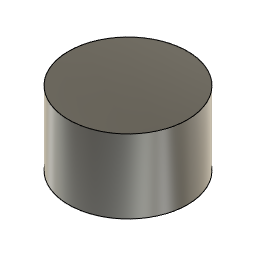
whole assembly (Autodesk Fusion 360 archive; units mm, degrees)
design "Knob"
Autodesk Fusion 360 part; units mm, degrees
(part 1 of 4)
sketch "Sketch1" plane through (0, 0, 0) normal (0, 0, 1) x (1, 0, 0)
  circle A0 centre (0, 0) radius 12.5
  circle A1 centre (0, 0) radius 3
  dimension "d1" = 25
  dimension "d2" = 6
  constraint coincident A0.centre A1.centre
  measures "d1" diameter of A0
  measures "d2" diameter of A1
extrude "Extrude1" add sketch "Sketch1" along normal blind 15.5 contours A0 | A1
extrude "Extrude2" cut sketch "Sketch1" along normal blind 11 contours A1

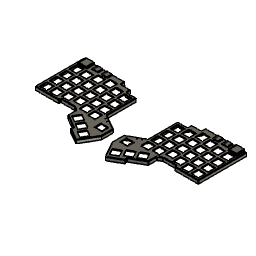
design "both_frame"
Autodesk Fusion 360 part; units mm, degrees
sketch "Sketch2" plane through (0, 0, 0) normal (0, 0, 1) x (1, 0, 0)
  line L0 (30.0248, 56.3298) -> (68.0248, 56.3298) construction
  line L1 (68.0248, 56.3298) -> (68.0248, -19.6702) construction
  line L2 (68.0248, -19.6702) -> (30.0248, -19.6702) construction
  line L3 (30.0248, -19.6702) -> (30.0248, 56.3298) construction
  line L4 (11.0248, 60.3298) -> (30.0248, 60.3298) construction
  line L5 (30.0248, 60.3298) -> (30.0248, -15.6702) construction
  line L6 (30.0248, -15.6702) -> (11.0248, -15.6702) construction
  line L7 (11.0248, -15.6702) -> (11.0248, 60.3298) construction
  line L8 (-7.9752, 64.3298) -> (11.0248, 64.3298) construction
  line L9 (11.0248, 64.3298) -> (11.0248, -11.6702) construction
  line L10 (11.0248, -11.6702) -> (-7.9752, -11.6702) construction
  line L11 (-7.9752, -11.6702) -> (-7.9752, 64.3298) construction
  line L12 (-26.9752, -18.6702) -> (-7.9752, -18.6702) construction
  line L13 (-7.9752, -18.6702) -> (-7.9752, 57.3298) construction
  line L14 (-7.9752, 57.3298) -> (-26.9752, 57.3298) construction
  line L15 (-26.9752, 57.3298) -> (-26.9752, -18.6702) construction
  line L16 (-45.9752, -21.6702) -> (-26.9752, -21.6702) construction
  line L17 (-26.9752, -21.6702) -> (-26.9752, 54.3298) construction
  line L18 (-26.9752, 54.3298) -> (-45.9752, 54.3298) construction
  line L19 (-45.9752, 54.3298) -> (-45.9752, -21.6702) construction
  line L20 (68.0248, 37.3298) -> (30.0248, 37.3298) construction
  line L21 (68.0248, 18.3298) -> (30.0248, 18.3298) construction
  line L22 (68.0248, -0.6702) -> (30.0248, -0.6702) construction
  line L23 (49.0248, 56.3298) -> (49.0248, -19.6702) construction
  line L24 (30.0248, 41.3298) -> (11.0248, 41.3298) construction
  line L25 (11.0248, 22.3298) -> (30.0248, 22.3298) construction
  line L26 (11.0248, 3.3298) -> (30.0248, 3.3298) construction
  line L27 (11.0248, 45.3298) -> (-7.9752, 45.3298) construction
  line L28 (-7.9752, 26.3298) -> (11.0248, 26.3298) construction
  line L29 (-7.9752, 7.3298) -> (11.0248, 7.3298) construction
  line L30 (-26.9752, 38.3298) -> (-7.9752, 38.3298) construction
  line L31 (-26.9752, 19.3298) -> (-7.9752, 19.3298) construction
  line L32 (-26.9752, 0.3298) -> (-7.9752, 0.3298) construction
  line L33 (-45.9752, 35.3298) -> (-26.9752, 35.3298) construction
  line L34 (-45.9752, 16.3298) -> (-26.9752, 16.3298) construction
  line L35 (-45.9752, -2.6702) -> (-26.9752, -2.6702) construction
  line L36 (-37.7979, -29.9811) -> (-21.3375, -20.4913) construction
  line L37 (-21.3375, -20.4913) -> (-11.8477, -36.9516) construction
  line L38 (-11.8477, -36.9516) -> (-28.3081, -46.4414) construction
  line L39 (-28.3081, -46.4414) -> (-37.7979, -29.9811) construction
  line L40 (-37.7979, -29.9811) -> (-54.2582, -39.4709) construction
  line L41 (-54.2582, -39.4709) -> (-44.7684, -55.9312) construction
  line L42 (-44.7684, -55.9312) -> (-28.3081, -46.4414) construction
  line L43 (-28.3081, -46.4414) -> (-37.7979, -29.9811) construction
  line L44 (-54.2582, -39.4709) -> (-70.7186, -48.9607) construction
  line L45 (-70.7186, -48.9607) -> (-58.8251, -69.5903) construction
  line L46 (-58.8251, -69.5903) -> (-42.3648, -60.1005) construction
  line L47 (-42.3648, -60.1005) -> (-54.2582, -39.4709) construction
  circle A0 centre (-63.2872, -26.2941) radius 12.5 construction
  line L48 (64.7748, 56.3298) -> (50.2748, 56.3298) construction
  line L49 (50.2748, 56.3298) -> (50.2748, 70.3298) construction
  line L50 (50.2748, 70.3298) -> (64.7748, 70.3298) construction
  line L51 (64.7748, 70.3298) -> (64.7748, 56.3298) construction
  line L52 (57.5248, 70.3298) -> (57.5248, 56.3298) construction
  line L53 (32.0248, 70.3298) -> (43.0248, 70.3298) construction
  line L54 (43.0248, 70.3298) -> (43.0248, 63.3298) construction
  line L55 (43.0248, 63.3298) -> (32.0248, 63.3298) construction
  line L56 (32.0248, 63.3298) -> (32.0248, 70.3298) construction
  line L57 (37.5248, 70.3298) -> (37.5248, 63.3298) construction
  line L58 (14.0248, 70.3298) -> (25.0248, 70.3298) construction
  line L59 (25.0248, 70.3298) -> (25.0248, 63.3298) construction
  line L60 (25.0248, 63.3298) -> (14.0248, 63.3298) construction
  line L61 (14.0248, 63.3298) -> (14.0248, 70.3298) construction
  line L62 (19.5248, 63.3298) -> (19.5248, 70.3298) construction
  line L63 (25.0248, 70.3298) -> (32.0248, 70.3298) construction
  line L64 (43.0248, 70.3298) -> (50.2748, 70.3298) construction
  line L65 (68.0248, 56.3298) -> (68.0248, 70.3298) construction
  line L66 (68.0248, 70.3298) -> (64.7748, 70.3298) construction
  line L67 (14.0248, 70.3298) -> (-7.9752, 70.3298) construction
  line L68 (-7.9752, 64.3298) -> (-7.9752, 70.3298) construction
  line L69 (-2.7791, -15.6702) -> (11.0248, -15.6702) construction
  line L70 (-11.8477, -36.9516) -> (-11.8477, -20.906) construction
  line L71 (-11.8477, -20.906) -> (-2.7791, -15.6702) construction
  line L72 (-42.3648, -60.1005) -> (-42.3648, -54.5455) construction
  line L73 (-70.7186, -48.9607) -> (-75.7872, -40.1691) construction
  line L74 (-75.7872, -40.1691) -> (-75.7872, -26.2941) construction
  line L75 (-69.5372, -15.4688) -> (-45.9752, -1.8653) construction
  line L76 (-45.9752, 54.3298) -> (-26.9752, 35.3298) construction
  line L77 (-45.9752, 35.3298) -> (-26.9752, 16.3298) construction
  line L78 (-45.9752, 16.3298) -> (-26.9752, -2.6702) construction
  line L79 (-45.9752, -2.6702) -> (-26.9752, -21.6702) construction
  line L80 (-26.9752, 0.3298) -> (-7.9752, -18.6702) construction
  line L81 (-26.9752, 19.3298) -> (-7.9752, 0.3298) construction
  line L82 (-7.9752, 7.3298) -> (11.0248, -11.6702) construction
  line L83 (11.0248, 3.3298) -> (30.0248, -15.6702) construction
  line L84 (11.0248, 22.3298) -> (30.0248, 3.3298) construction
  line L85 (-7.9752, 26.3298) -> (11.0248, 7.3298) construction
  line L86 (-26.9752, 57.3298) -> (-7.9752, 38.3298) construction
  line L87 (-26.9752, 38.3298) -> (-7.9752, 19.3298) construction
  line L88 (11.0248, 60.3298) -> (30.0248, 41.3298) construction
  line L89 (-7.9752, 64.3298) -> (11.0248, 45.3298) construction
  line L90 (-7.9752, 45.3298) -> (11.0248, 26.3298) construction
  line L91 (11.0248, 41.3298) -> (30.0248, 22.3298) construction
  line L92 (30.0248, 56.3298) -> (49.0248, 37.3298) construction
  line L93 (49.0248, 56.3298) -> (68.0248, 37.3298) construction
  line L94 (30.0248, 37.3298) -> (49.0248, 18.3298) construction
  line L95 (49.0248, 37.3298) -> (68.0248, 18.3298) construction
  line L96 (49.0248, 18.3298) -> (68.0248, -0.6702) construction
  line L97 (30.0248, 18.3298) -> (49.0248, -0.6702) construction
  line L98 (30.0248, -0.6702) -> (49.0248, -19.6702) construction
  line L99 (49.0248, -0.6702) -> (68.0248, -19.6702) construction
  line L100 (-28.3081, -46.4414) -> (-21.3375, -20.4913) construction
  line L101 (-44.7684, -55.9312) -> (-37.7979, -29.9811) construction
  line L102 (-58.8251, -69.5903) -> (-54.2582, -39.4709) construction
  line L103 (-75.7872, -26.2941) -> (-75.7872, -19.0772) construction
  line L104 (-75.7872, -19.0772) -> (-69.5372, -15.4688) construction
  line L105 (68.0248, 70.3298) -> (68.0248, -19.6702)
  line L106 (30.0248, -19.6702) -> (68.0248, -19.6702)
  line L107 (30.0248, -19.6702) -> (30.0248, -15.6702)
  line L108 (11.0248, -15.6702) -> (30.0248, -15.6702)
  line L109 (11.0248, -15.6702) -> (-2.7791, -15.6702)
  line L110 (-2.7791, -15.6702) -> (-11.8477, -20.906)
  line L111 (-11.8477, -36.9516) -> (-11.8477, -20.906)
  line L112 (-11.8477, -36.9516) -> (-44.7684, -55.9312)
  line L113 (-42.3648, -60.1005) -> (-44.7684, -55.9312)
  line L114 (-42.3648, -60.1005) -> (-58.8251, -69.5903)
  line L115 (-58.8251, -69.5903) -> (-75.7872, -40.1691)
  line L116 (-75.7872, -40.1691) -> (-75.7872, -19.0772)
  line L117 (-75.7872, -19.0772) -> (-45.9752, -1.8653)
  line L118 (-45.9752, -1.8653) -> (-45.9752, 54.3298)
  line L119 (-45.9752, 54.3298) -> (-26.9752, 54.3298)
  line L120 (-26.9752, 54.3298) -> (-26.9752, 57.3298)
  line L121 (-26.9752, 57.3298) -> (-7.9752, 57.3298)
  line L122 (-7.9752, 57.3298) -> (-7.9752, 70.3298)
  line L123 (-7.9752, 70.3298) -> (68.0248, 70.3298)
  line L124 (-29.3752, 37.7298) -> (-43.5752, 37.7298)
  line L125 (-43.5752, 37.7298) -> (-43.5752, 51.9298)
  line L126 (-43.5752, 51.9298) -> (-29.3752, 51.9298)
  line L127 (-29.3752, 51.9298) -> (-29.3752, 37.7298)
  line L128 (-29.3752, 37.7298) -> (-43.5752, 51.9298) construction
  line L129 (-43.5752, 37.7298) -> (-29.3752, 51.9298) construction
  line L130 (-10.3752, 40.7298) -> (-24.5752, 40.7298)
  line L131 (-24.5752, 40.7298) -> (-24.5752, 54.9298)
  line L132 (-24.5752, 54.9298) -> (-10.3752, 54.9298)
  line L133 (-10.3752, 54.9298) -> (-10.3752, 40.7298)
  line L134 (-10.3752, 40.7298) -> (-24.5752, 54.9298) construction
  line L135 (-24.5752, 40.7298) -> (-10.3752, 54.9298) construction
  line L136 (8.6248, 47.7298) -> (-5.5752, 47.7298)
  line L137 (-5.5752, 47.7298) -> (-5.5752, 61.9298)
  line L138 (-5.5752, 61.9298) -> (8.6248, 61.9298)
  line L139 (8.6248, 61.9298) -> (8.6248, 47.7298)
  line L140 (8.6248, 47.7298) -> (-5.5752, 61.9298) construction
  line L141 (-5.5752, 47.7298) -> (8.6248, 61.9298) construction
  line L142 (27.6248, 43.7298) -> (13.4248, 43.7298)
  line L143 (13.4248, 43.7298) -> (13.4248, 57.9298)
  line L144 (13.4248, 57.9298) -> (27.6248, 57.9298)
  line L145 (27.6248, 57.9298) -> (27.6248, 43.7298)
  line L146 (27.6248, 43.7298) -> (13.4248, 57.9298) construction
  line L147 (13.4248, 43.7298) -> (27.6248, 57.9298) construction
  line L148 (46.6248, 39.7298) -> (32.4248, 39.7298)
  line L149 (32.4248, 39.7298) -> (32.4248, 53.9298)
  line L150 (32.4248, 53.9298) -> (46.6248, 53.9298)
  line L151 (46.6248, 53.9298) -> (46.6248, 39.7298)
  line L152 (46.6248, 39.7298) -> (32.4248, 53.9298) construction
  line L153 (32.4248, 39.7298) -> (46.6248, 53.9298) construction
  line L154 (65.6248, 39.7298) -> (51.4248, 39.7298)
  line L155 (51.4248, 39.7298) -> (51.4248, 53.9298)
  line L156 (51.4248, 53.9298) -> (65.6248, 53.9298)
  line L157 (65.6248, 53.9298) -> (65.6248, 39.7298)
  line L158 (65.6248, 39.7298) -> (51.4248, 53.9298) construction
  line L159 (51.4248, 39.7298) -> (65.6248, 53.9298) construction
  line L160 (65.6248, 20.7298) -> (51.4248, 20.7298)
  line L161 (51.4248, 20.7298) -> (51.4248, 34.9298)
  line L162 (51.4248, 34.9298) -> (65.6248, 34.9298)
  line L163 (65.6248, 34.9298) -> (65.6248, 20.7298)
  line L164 (65.6248, 20.7298) -> (51.4248, 34.9298) construction
  line L165 (51.4248, 20.7298) -> (65.6248, 34.9298) construction
  line L166 (46.6248, 20.7298) -> (32.4248, 20.7298)
  line L167 (32.4248, 20.7298) -> (32.4248, 34.9298)
  line L168 (32.4248, 34.9298) -> (46.6248, 34.9298)
  line L169 (46.6248, 34.9298) -> (46.6248, 20.7298)
  line L170 (46.6248, 20.7298) -> (32.4248, 34.9298) construction
  line L171 (32.4248, 20.7298) -> (46.6248, 34.9298) construction
  line L172 (65.6248, 1.7298) -> (51.4248, 1.7298)
  line L173 (51.4248, 1.7298) -> (51.4248, 15.9298)
  line L174 (51.4248, 15.9298) -> (65.6248, 15.9298)
  line L175 (65.6248, 15.9298) -> (65.6248, 1.7298)
  line L176 (65.6248, 1.7298) -> (51.4248, 15.9298) construction
  line L177 (51.4248, 1.7298) -> (65.6248, 15.9298) construction
  line L178 (46.6248, 1.7298) -> (32.4248, 1.7298)
  line L179 (32.4248, 1.7298) -> (32.4248, 15.9298)
  line L180 (32.4248, 15.9298) -> (46.6248, 15.9298)
  line L181 (46.6248, 15.9298) -> (46.6248, 1.7298)
  line L182 (46.6248, 1.7298) -> (32.4248, 15.9298) construction
  line L183 (32.4248, 1.7298) -> (46.6248, 15.9298) construction
  line L184 (46.6248, -17.2702) -> (32.4248, -17.2702)
  line L185 (32.4248, -17.2702) -> (32.4248, -3.0702)
  line L186 (32.4248, -3.0702) -> (46.6248, -3.0702)
  line L187 (46.6248, -3.0702) -> (46.6248, -17.2702)
  line L188 (46.6248, -17.2702) -> (32.4248, -3.0702) construction
  line L189 (32.4248, -17.2702) -> (46.6248, -3.0702) construction
  line L190 (65.6248, -17.2702) -> (51.4248, -17.2702)
  line L191 (51.4248, -17.2702) -> (51.4248, -3.0702)
  line L192 (51.4248, -3.0702) -> (65.6248, -3.0702)
  line L193 (65.6248, -3.0702) -> (65.6248, -17.2702)
  line L194 (65.6248, -17.2702) -> (51.4248, -3.0702) construction
  line L195 (51.4248, -17.2702) -> (65.6248, -3.0702) construction
  line L196 (27.6248, -13.2702) -> (13.4248, -13.2702)
  line L197 (13.4248, -13.2702) -> (13.4248, 0.9298)
  line L198 (13.4248, 0.9298) -> (27.6248, 0.9298)
  line L199 (27.6248, 0.9298) -> (27.6248, -13.2702)
  line L200 (27.6248, -13.2702) -> (13.4248, 0.9298) construction
  line L201 (13.4248, -13.2702) -> (27.6248, 0.9298) construction
  line L202 (8.6248, -9.2702) -> (-5.5752, -9.2702)
  line L203 (-5.5752, -9.2702) -> (-5.5752, 4.9298)
  line L204 (-5.5752, 4.9298) -> (8.6248, 4.9298)
  line L205 (8.6248, 4.9298) -> (8.6248, -9.2702)
  line L206 (8.6248, -9.2702) -> (-5.5752, 4.9298) construction
  line L207 (-5.5752, -9.2702) -> (8.6248, 4.9298) construction
  line L208 (27.6248, 5.7298) -> (13.4248, 5.7298)
  line L209 (13.4248, 5.7298) -> (13.4248, 19.9298)
  line L210 (13.4248, 19.9298) -> (27.6248, 19.9298)
  line L211 (27.6248, 19.9298) -> (27.6248, 5.7298)
  line L212 (27.6248, 5.7298) -> (13.4248, 19.9298) construction
  line L213 (13.4248, 5.7298) -> (27.6248, 19.9298) construction
  line L214 (8.6248, 9.7298) -> (-5.5752, 9.7298)
  line L215 (-5.5752, 9.7298) -> (-5.5752, 23.9298)
  line L216 (-5.5752, 23.9298) -> (8.6248, 23.9298)
  line L217 (8.6248, 23.9298) -> (8.6248, 9.7298)
  line L218 (8.6248, 9.7298) -> (-5.5752, 23.9298) construction
  line L219 (-5.5752, 9.7298) -> (8.6248, 23.9298) construction
  line L220 (27.6248, 24.7298) -> (13.4248, 24.7298)
  line L221 (13.4248, 24.7298) -> (13.4248, 38.9298)
  line L222 (13.4248, 38.9298) -> (27.6248, 38.9298)
  line L223 (27.6248, 38.9298) -> (27.6248, 24.7298)
  line L224 (27.6248, 24.7298) -> (13.4248, 38.9298) construction
  line L225 (13.4248, 24.7298) -> (27.6248, 38.9298) construction
  line L226 (8.6248, 28.7298) -> (-5.5752, 28.7298)
  line L227 (-5.5752, 28.7298) -> (-5.5752, 42.9298)
  line L228 (-5.5752, 42.9298) -> (8.6248, 42.9298)
  line L229 (8.6248, 42.9298) -> (8.6248, 28.7298)
  line L230 (8.6248, 28.7298) -> (-5.5752, 42.9298) construction
  line L231 (-5.5752, 28.7298) -> (8.6248, 42.9298) construction
  line L232 (-10.3752, 21.7298) -> (-24.5752, 21.7298)
  line L233 (-24.5752, 21.7298) -> (-24.5752, 35.9298)
  line L234 (-24.5752, 35.9298) -> (-10.3752, 35.9298)
  line L235 (-10.3752, 35.9298) -> (-10.3752, 21.7298)
  line L236 (-10.3752, 21.7298) -> (-24.5752, 35.9298) construction
  line L237 (-24.5752, 21.7298) -> (-10.3752, 35.9298) construction
  line L238 (-29.3752, 18.7298) -> (-43.5752, 18.7298)
  line L239 (-43.5752, 18.7298) -> (-43.5752, 32.9298)
  line L240 (-43.5752, 32.9298) -> (-29.3752, 32.9298)
  line L241 (-29.3752, 32.9298) -> (-29.3752, 18.7298)
  line L242 (-29.3752, 18.7298) -> (-43.5752, 32.9298) construction
  line L243 (-43.5752, 18.7298) -> (-29.3752, 32.9298) construction
  line L244 (-10.3752, 2.7298) -> (-24.5752, 2.7298)
  line L245 (-24.5752, 2.7298) -> (-24.5752, 16.9298)
  line L246 (-24.5752, 16.9298) -> (-10.3752, 16.9298)
  line L247 (-10.3752, 16.9298) -> (-10.3752, 2.7298)
  line L248 (-10.3752, 2.7298) -> (-24.5752, 16.9298) construction
  line L249 (-24.5752, 2.7298) -> (-10.3752, 16.9298) construction
  line L250 (-10.3752, -16.2702) -> (-24.5752, -16.2702)
  line L251 (-24.5752, -16.2702) -> (-24.5752, -2.0702)
  line L252 (-24.5752, -2.0702) -> (-10.3752, -2.0702)
  line L253 (-10.3752, -2.0702) -> (-10.3752, -16.2702)
  line L254 (-10.3752, -16.2702) -> (-24.5752, -2.0702) construction
  line L255 (-24.5752, -16.2702) -> (-10.3752, -2.0702) construction
  line L256 (-29.3752, -0.2702) -> (-43.5752, -0.2702)
  line L257 (-43.5752, -0.2702) -> (-43.5752, 13.9298)
  line L258 (-43.5752, 13.9298) -> (-29.3752, 13.9298)
  line L259 (-29.3752, 13.9298) -> (-29.3752, -0.2702)
  line L260 (-29.3752, -0.2702) -> (-43.5752, 13.9298) construction
  line L261 (-43.5752, -0.2702) -> (-29.3752, 13.9298) construction
  line L262 (-29.3752, -19.2702) -> (-43.5752, -19.2702)
  line L263 (-43.5752, -19.2702) -> (-43.5752, -5.0702)
  line L264 (-43.5752, -5.0702) -> (-29.3752, -5.0702)
  line L265 (-29.3752, -5.0702) -> (-29.3752, -19.2702)
  line L266 (-29.3752, -19.2702) -> (-43.5752, -5.0702) construction
  line L267 (-43.5752, -19.2702) -> (-29.3752, -5.0702) construction
  line L268 (-15.1256, -36.0711) -> (-27.4276, -43.1635)
  line L269 (-27.4276, -43.1635) -> (-34.52, -30.8616)
  line L270 (-34.52, -30.8616) -> (-22.218, -23.7692)
  line L271 (-22.218, -23.7692) -> (-15.1256, -36.0711)
  line L272 (-15.1256, -36.0711) -> (-34.52, -30.8616) construction
  line L273 (-27.4276, -43.1635) -> (-22.218, -23.7692) construction
  line L274 (-31.586, -45.5609) -> (-43.8879, -52.6533)
  line L275 (-43.8879, -52.6533) -> (-50.9803, -40.3514)
  line L276 (-50.9803, -40.3514) -> (-38.6784, -33.259)
  line L277 (-38.6784, -33.259) -> (-31.586, -45.5609)
  line L278 (-31.586, -45.5609) -> (-50.9803, -40.3514) construction
  line L279 (-43.8879, -52.6533) -> (-38.6784, -33.259) construction
  line L280 (-46.8445, -57.1354) -> (-59.1465, -64.2278)
  line L281 (-59.1465, -64.2278) -> (-66.2388, -51.9258)
  line L282 (-66.2388, -51.9258) -> (-53.9369, -44.8334)
  line L283 (-53.9369, -44.8334) -> (-46.8445, -57.1354)
  line L284 (-46.8445, -57.1354) -> (-66.2388, -51.9258) construction
  line L285 (-59.1465, -64.2278) -> (-53.9369, -44.8334) construction
  line L286 (-57.0872, -32.3441) -> (-69.4872, -32.3441)
  line L287 (-69.4872, -32.3441) -> (-69.4872, -20.2441)
  line L288 (-69.4872, -20.2441) -> (-57.0872, -20.2441)
  line L289 (-57.0872, -20.2441) -> (-57.0872, -32.3441)
  line L290 (-57.0872, -32.3441) -> (-69.4872, -20.2441) construction
  line L291 (-69.4872, -32.3441) -> (-57.0872, -20.2441) construction
  point P0 (-36.4752, 44.8298)
  point P1 (-17.4752, 47.8298)
  point P2 (1.5248, 54.8298)
  point P3 (20.5248, 50.8298)
  point P4 (39.5248, 46.8298)
  point P5 (58.5248, 46.8298)
  point P6 (58.5248, 27.8298)
  point P7 (39.5248, 27.8298)
  point P8 (58.5248, 8.8298)
  point P9 (39.5248, 8.8298)
  point P10 (39.5248, -10.1702)
  point P11 (58.5248, -10.1702)
  point P12 (20.5248, -6.1702)
  point P13 (1.5248, -2.1702)
  point P14 (20.5248, 12.8298)
  point P15 (1.5248, 16.8298)
  point P16 (20.5248, 31.8298)
  point P17 (1.5248, 35.8298)
  point P18 (-17.4752, 28.8298)
  point P19 (-36.4752, 25.8298)
  point P20 (-17.4752, 9.8298)
  point P21 (-17.4752, -9.1702)
  point P22 (-36.4752, 6.8298)
  point P23 (-36.4752, -12.1702)
  point P24 (-24.8228, -33.4664)
  point P25 (-41.2831, -42.9562)
  point P26 (-56.5417, -54.5306)
  point P27 (-63.2872, -26.2941)
  dimension "d1" = 76
  dimension "d2" = 38
  dimension "d3" = 76
  dimension "d4" = 4
  dimension "d5" = 19
  dimension "d6" = 19
  dimension "d7" = 76
  dimension "d8" = 19
  dimension "d9" = 19
  dimension "d10" = 76
  dimension "d11" = 76
  dimension "d12" = 4
  dimension "d13" = 7
  dimension "d14" = 3
  dimension "d15" = 19
  dimension "d16" = 19
  dimension "d17" = 19
  dimension "d18" = 19
  dimension "d19" = 19
  dimension "d20" = 19
  dimension "d21" = 19
  dimension "d22" = 19
  dimension "d23" = 19
  dimension "d24" = 19
  dimension "d25" = 19
  dimension "d26" = 19
  dimension "d27" = 19
  dimension "d28" = 19
  dimension "d29" = 19
  dimension "d31" = 19
  dimension "d33" = 23.8125
  dimension "d35" = 25
  dimension "d36" = 14
  dimension "d37" = 14.5
  dimension "d38" = 20
  dimension "d39" = 11
  dimension "d40" = 7
  dimension "d41" = 18
  dimension "d42" = 3
  dimension "d43" = 3
  dimension "d44" = 150
  dimension "d45" = 60
  dimension "d79" = 14.2
  dimension "d111" = 12.4
  dimension "d112" = 12.1
  constraint horizontal L0
  constraint vertical L1
  constraint horizontal L2
  constraint vertical L3
  constraint horizontal L4
  constraint vertical L5
  constraint horizontal L6
  constraint vertical L7
  constraint coincident L3 L5.end
  constraint horizontal L8
  constraint vertical L9
  constraint horizontal L10
  constraint vertical L11
  constraint coincident L7 L9.end
  constraint horizontal L12
  constraint vertical L13
  constraint horizontal L14
  constraint vertical L15
  constraint coincident L11 L13.end
  constraint horizontal L16
  constraint vertical L17
  constraint horizontal L18
  constraint vertical L19
  constraint coincident L15 L17.end
  constraint coincident L1 L20.start
  constraint coincident L5 L20.end
  constraint perpendicular L5 L20
  constraint coincident L1 L21.start
  constraint coincident L5 L21.end
  constraint coincident L1 L22.start
  constraint coincident L5 L22.end
  constraint coincident L0 L23.start
  constraint midpoint L2 L23.end
  constraint coincident L5 L24.start
  constraint coincident L7 L24.end
  constraint coincident L7 L25.start
  constraint coincident L3 L25.end
  constraint coincident L9 L26.start
  constraint coincident L5 L26.end
  constraint coincident L7 L27.start
  constraint coincident L11 L27.end
  constraint coincident L13 L28.start
  constraint coincident L7 L28.end
  constraint coincident L11 L29.start
  constraint coincident L7 L29.end
  constraint coincident L15 L30.start
  constraint coincident L11 L30.end
  constraint coincident L17 L31.start
  constraint coincident L13 L31.end
  constraint coincident L17 L32.start
  constraint coincident L13 L32.end
  constraint coincident L19 L33.start
  constraint coincident L15 L33.end
  constraint coincident L19 L34.start
  constraint coincident L15 L34.end
  constraint coincident L19 L35.start
  constraint coincident L15 L35.end
  constraint vertical L23
  constraint horizontal L21
  constraint horizontal L22
  constraint horizontal L24
  constraint horizontal L25
  constraint horizontal L26
  constraint horizontal L29
  constraint horizontal L28
  constraint horizontal L27
  constraint horizontal L30
  constraint horizontal L31
  constraint horizontal L32
  constraint horizontal L34
  constraint horizontal L35
  constraint horizontal L33
  constraint equal L36 L37
  constraint equal L40 L43
  constraint equal L36 L40
  constraint equal L36 L44
  constraint perpendicular L36 L37
  constraint perpendicular L40 L43
  constraint perpendicular L37 L38
  constraint perpendicular L38 L43
  constraint perpendicular L36 L39
  constraint perpendicular L39 L42
  constraint perpendicular L40 L41
  constraint perpendicular L41 L44
  constraint perpendicular L44 L45
  constraint perpendicular L45 L46
  constraint perpendicular L46 L47
  constraint horizontal L48
  constraint vertical L49
  constraint horizontal L50
  constraint vertical L51
  constraint coincident L0 L48.start
  constraint midpoint L50 L52.start
  constraint midpoint L48 L52.end
  constraint horizontal L53
  constraint vertical L54
  constraint horizontal L55
  constraint vertical L56
  constraint collinear L50 L53
  constraint midpoint L53 L57.start
  constraint midpoint L55 L57.end
  constraint horizontal L58
  constraint vertical L59
  constraint horizontal L60
  constraint vertical L61
  constraint equal L56 L61
  constraint equal L53 L58
  constraint collinear L53 L58
  constraint midpoint L60 L62.start
  constraint midpoint L58 L62.end
  constraint perpendicular L0 L65
  constraint perpendicular L51 L66
  constraint perpendicular L61 L67
  constraint vertical L68
  constraint horizontal L69
  constraint vertical L70
  constraint coincident L42 L72.end
  constraint vertical L72
  constraint coincident L12.end L71
  constraint perpendicular L44 L73
  constraint coincident A0 L74.end
  constraint vertical L74
  constraint tangent A0 L74
  constraint coincident A0 L75.start
  constraint coincident L19 L75.end
  constraint tangent A0 L75
  constraint midpoint L20 L92.end
  constraint midpoint L21 L94.end
  constraint midpoint L22 L97.end
  constraint tangent A0 L103
  constraint collinear L75 L104
  constraint horizontal L124
  constraint perpendicular L124 L125
  constraint parallel L124 L126
  constraint parallel L125 L127
  constraint coincident L128 P0
  constraint coincident L129 P0
  constraint coincident L76 L124.start
  constraint midpoint L76 P0
  constraint horizontal L130
  constraint perpendicular L130 L131
  constraint parallel L130 L132
  constraint parallel L131 L133
  constraint coincident L134 P1
  constraint coincident L135 P1
  constraint coincident L86 L130.start
  constraint midpoint L86 P1
  constraint horizontal L136
  constraint perpendicular L136 L137
  constraint parallel L136 L138
  constraint parallel L137 L139
  constraint coincident L140 P2
  constraint coincident L141 P2
  constraint coincident L89 L136.start
  constraint midpoint L89 P2
  constraint horizontal L142
  constraint perpendicular L142 L143
  constraint parallel L142 L144
  constraint parallel L143 L145
  constraint coincident L146 P3
  constraint coincident L147 P3
  constraint coincident L88 L142.start
  constraint midpoint L88 P3
  constraint horizontal L148
  constraint perpendicular L148 L149
  constraint parallel L148 L150
  constraint parallel L149 L151
  constraint coincident L152 P4
  constraint coincident L153 P4
  constraint coincident L92 L148.start
  constraint midpoint L92 P4
  constraint horizontal L154
  constraint perpendicular L154 L155
  constraint parallel L154 L156
  constraint parallel L155 L157
  constraint coincident L158 P5
  constraint coincident L159 P5
  constraint coincident L93 L154.start
  constraint midpoint L93 P5
  constraint horizontal L160
  constraint perpendicular L160 L161
  constraint parallel L160 L162
  constraint parallel L161 L163
  constraint coincident L164 P6
  constraint coincident L165 P6
  constraint coincident L95 L160.start
  constraint midpoint L95 P6
  constraint horizontal L166
  constraint perpendicular L166 L167
  constraint parallel L166 L168
  constraint parallel L167 L169
  constraint coincident L170 P7
  constraint coincident L171 P7
  constraint coincident L94 L166.start
  constraint midpoint L94 P7
  constraint horizontal L172
  constraint perpendicular L172 L173
  constraint parallel L172 L174
  constraint parallel L173 L175
  constraint coincident L176 P8
  constraint coincident L177 P8
  constraint coincident L96 L172.start
  constraint midpoint L96 P8
  constraint horizontal L178
  constraint perpendicular L178 L179
  constraint parallel L178 L180
  constraint parallel L179 L181
  constraint coincident L182 P9
  constraint coincident L183 P9
  constraint coincident L97 L178.start
  constraint midpoint L97 P9
  constraint horizontal L184
  constraint perpendicular L184 L185
  constraint parallel L184 L186
  constraint parallel L185 L187
  constraint coincident L188 P10
  constraint coincident L189 P10
  constraint coincident L98 L184.start
  constraint midpoint L98 P10
  constraint horizontal L190
  constraint perpendicular L190 L191
  constraint parallel L190 L192
  constraint parallel L191 L193
  constraint coincident L194 P11
  constraint coincident L195 P11
  constraint coincident L99 L190.start
  constraint midpoint L99 P11
  constraint horizontal L196
  constraint perpendicular L196 L197
  constraint parallel L196 L198
  constraint parallel L197 L199
  constraint coincident L200 P12
  constraint coincident L201 P12
  constraint coincident L83 L196.start
  constraint midpoint L83 P12
  constraint horizontal L202
  constraint perpendicular L202 L203
  constraint parallel L202 L204
  constraint parallel L203 L205
  constraint coincident L206 P13
  constraint coincident L207 P13
  constraint coincident L82 L202.start
  constraint midpoint L82 P13
  constraint horizontal L208
  constraint perpendicular L208 L209
  constraint parallel L208 L210
  constraint parallel L209 L211
  constraint coincident L212 P14
  constraint coincident L213 P14
  constraint coincident L84 L208.start
  constraint midpoint L84 P14
  constraint horizontal L214
  constraint perpendicular L214 L215
  constraint parallel L214 L216
  constraint parallel L215 L217
  constraint coincident L218 P15
  constraint coincident L219 P15
  constraint coincident L85 L214.start
  constraint midpoint L85 P15
  constraint horizontal L220
  constraint perpendicular L220 L221
  constraint parallel L220 L222
  constraint parallel L221 L223
  constraint coincident L224 P16
  constraint coincident L225 P16
  constraint coincident L91 L220.start
  constraint midpoint L91 P16
  constraint horizontal L226
  constraint perpendicular L226 L227
  constraint parallel L226 L228
  constraint parallel L227 L229
  constraint coincident L230 P17
  constraint coincident L231 P17
  constraint coincident L90 L226.start
  constraint midpoint L90 P17
  constraint horizontal L232
  constraint perpendicular L232 L233
  constraint parallel L232 L234
  constraint parallel L233 L235
  constraint coincident L236 P18
  constraint coincident L237 P18
  constraint coincident L87 L232.start
  constraint midpoint L87 P18
  constraint horizontal L238
  constraint perpendicular L238 L239
  constraint parallel L238 L240
  constraint parallel L239 L241
  constraint coincident L242 P19
  constraint coincident L243 P19
  constraint coincident L77 L238.start
  constraint midpoint L77 P19
  constraint horizontal L244
  constraint perpendicular L244 L245
  constraint parallel L244 L246
  constraint parallel L245 L247
  constraint coincident L248 P20
  constraint coincident L249 P20
  constraint coincident L81 L244.start
  constraint midpoint L81 P20
  constraint horizontal L250
  constraint perpendicular L250 L251
  constraint parallel L250 L252
  constraint parallel L251 L253
  constraint coincident L254 P21
  constraint coincident L255 P21
  constraint coincident L80 L250.start
  constraint midpoint L80 P21
  constraint horizontal L256
  constraint perpendicular L256 L257
  constraint parallel L256 L258
  constraint parallel L257 L259
  constraint coincident L260 P22
  constraint coincident L261 P22
  constraint coincident L78 L256.start
  constraint midpoint L78 P22
  constraint horizontal L262
  constraint perpendicular L262 L263
  constraint parallel L262 L264
  constraint parallel L263 L265
  constraint coincident L266 P23
  constraint coincident L267 P23
  constraint coincident L79 L262.start
  constraint midpoint L79 P23
  constraint perpendicular L268 L269
  constraint parallel L268 L270
  constraint parallel L269 L271
  constraint coincident L272 P24
  constraint coincident L273 P24
  constraint midpoint L100 P24
  constraint perpendicular L274 L275
  constraint parallel L274 L276
  constraint parallel L275 L277
  constraint coincident L278 P25
  constraint coincident L279 P25
  constraint midpoint L101 P25
  constraint parallel L280 L282
  constraint parallel L281 L283
  constraint coincident L284 P26
  constraint coincident L285 P26
  constraint midpoint L102 P26
  constraint collinear L101 L279
  constraint collinear L100 L273
  constraint perpendicular L284 L285
  constraint perpendicular L101 L278
  constraint perpendicular L100 L272
  constraint equal L126 L132
  constraint equal L126 L138
  constraint equal L126 L144
  constraint equal L126 L150
  constraint equal L126 L168
  constraint equal L126 L162
  constraint equal L126 L156
  constraint equal L126 L240
  constraint equal L126 L234
  constraint equal L126 L228
  constraint equal L126 L222
  constraint equal L126 L210
  constraint equal L126 L216
  constraint equal L126 L246
  constraint equal L126 L180
  constraint equal L126 L174
  constraint equal L126 L192
  constraint equal L126 L186
  constraint equal L126 L198
  constraint equal L126 L204
  constraint equal L126 L252
  constraint equal L126 L258
  constraint equal L126 L264
  constraint equal L126 L270
  constraint equal L126 L276
  constraint parallel L275 L283
  constraint parallel L276 L282
  constraint equal L126 L282
  constraint horizontal L286
  constraint perpendicular L286 L287
  constraint parallel L286 L288
  constraint parallel L287 L289
  constraint coincident L290 P27
  constraint coincident L291 P27
  constraint coincident P27 A0.centre
  measures "d1" distance of L0.end L1.end
  measures "d2" distance of L0.start L0.end
  measures "d3" distance of L4 L6
  measures "d4" distance of L2 L6
  measures "d5" distance of L4.start L4.end
  measures "d6" distance of L8.start L8.end
  measures "d7" distance of L8 L10
  measures "d8" distance of L13.end L14.end
  measures "d9" distance of L17.end L18.end
  measures "d10" distance of L12 L14
  measures "d11" distance of L16 L18
  measures "d12" distance of L6 L10
  measures "d13" distance of L10 L12
  measures "d14" distance of L12 L16
  measures "d15" distance of L0 L20
  measures "d16" distance of L20 L21
  measures "d17" distance of L21 L22
  measures "d18" distance of L4 L24
  measures "d19" distance of L24 L25
  measures "d20" distance of L25 L26
  measures "d21" distance of L8 L27
  measures "d22" distance of L27 L28
  measures "d23" distance of L28 L29
  measures "d24" distance of L14 L30
  measures "d25" distance of L30 L31
  measures "d26" distance of L31 L32
  measures "d27" distance of L18 L33
  measures "d28" distance of L33 L34
  measures "d29" distance of L34 L35
  measures "d31" distance of L36.start L36.end
  measures "d33" distance of L44.end L45.end
  measures "d35" diameter of A0
  measures "d36" distance of L48.start L50.end
  measures "d37" distance of L49.end L50.end
  measures "d38" distance of L52 L57
  measures "d39" distance of L53.start L53.end
  measures "d40" distance of L53.start L55.end
  measures "d41" distance of L57 L62
  measures "d42" distance of L4 L60
  measures "d43" distance of L9 L61
  measures "d44" angle of L69 L71
  measures "d45" angle of L19 L75
  measures "d79" distance of L125.end L126.end
  measures "d111" distance of L287.end L288.end
  measures "d112" distance of L286.end L287.end
extrude "Extrude3" add sketch "Sketch2" along normal blind 2.5 makes body 1
sketch "Sketch6" plane through (0, 0, 0) normal (0, 0, -1) x (1, 0, 0)
  line L0 (-10.3752, -16.9298) -> (-24.5752, -16.9298)
  line L1 (-24.5752, -16.9298) -> (-24.5752, -2.7298)
  line L2 (-24.5752, -2.7298) -> (-10.3752, -2.7298)
  line L3 (-10.3752, -2.7298) -> (-10.3752, -16.9298)
  line L4 (-10.3752, 2.0702) -> (-24.5752, 2.0702)
  line L5 (-24.5752, 2.0702) -> (-24.5752, 16.2702)
  line L6 (-24.5752, 16.2702) -> (-10.3752, 16.2702)
  line L7 (-10.3752, 16.2702) -> (-10.3752, 2.0702)
  line L8 (-29.3752, 5.0702) -> (-43.5752, 5.0702)
  line L9 (-43.5752, 5.0702) -> (-43.5752, 19.2702)
  line L10 (-43.5752, 19.2702) -> (-29.3752, 19.2702)
  line L11 (-29.3752, 19.2702) -> (-29.3752, 5.0702)
  line L12 (-29.3752, -32.9298) -> (-43.5752, -32.9298)
  line L13 (-43.5752, -32.9298) -> (-43.5752, -18.7298)
  line L14 (-43.5752, -18.7298) -> (-29.3752, -18.7298)
  line L15 (-29.3752, -18.7298) -> (-29.3752, -32.9298)
  line L16 (-29.3752, -13.9298) -> (-43.5752, -13.9298)
  line L17 (-43.5752, -13.9298) -> (-43.5752, 0.2702)
  line L18 (-43.5752, 0.2702) -> (-29.3752, 0.2702)
  line L19 (-29.3752, 0.2702) -> (-29.3752, -13.9298)
  line L20 (-10.3752, -35.9298) -> (-24.5752, -35.9298)
  line L21 (-24.5752, -35.9298) -> (-24.5752, -21.7298)
  line L22 (-24.5752, -21.7298) -> (-10.3752, -21.7298)
  line L23 (-10.3752, -21.7298) -> (-10.3752, -35.9298)
  line L24 (8.6248, -42.9298) -> (-5.5752, -42.9298)
  line L25 (-5.5752, -42.9298) -> (-5.5752, -28.7298)
  line L26 (-5.5752, -28.7298) -> (8.6248, -28.7298)
  line L27 (8.6248, -28.7298) -> (8.6248, -42.9298)
  line L28 (27.6248, -38.9298) -> (13.4248, -38.9298)
  line L29 (13.4248, -38.9298) -> (13.4248, -24.7298)
  line L30 (13.4248, -24.7298) -> (27.6248, -24.7298)
  line L31 (27.6248, -24.7298) -> (27.6248, -38.9298)
  line L32 (8.6248, -23.9298) -> (-5.5752, -23.9298)
  line L33 (-5.5752, -23.9298) -> (-5.5752, -9.7298)
  line L34 (-5.5752, -9.7298) -> (8.6248, -9.7298)
  line L35 (8.6248, -9.7298) -> (8.6248, -23.9298)
  line L36 (27.6248, -19.9298) -> (13.4248, -19.9298)
  line L37 (13.4248, -19.9298) -> (13.4248, -5.7298)
  line L38 (13.4248, -5.7298) -> (27.6248, -5.7298)
  line L39 (27.6248, -5.7298) -> (27.6248, -19.9298)
  line L40 (8.6248, -4.9298) -> (-5.5752, -4.9298)
  line L41 (-5.5752, -4.9298) -> (-5.5752, 9.2702)
  line L42 (-5.5752, 9.2702) -> (8.6248, 9.2702)
  line L43 (8.6248, 9.2702) -> (8.6248, -4.9298)
  line L44 (27.6248, -0.9298) -> (13.4248, -0.9298)
  line L45 (13.4248, -0.9298) -> (13.4248, 13.2702)
  line L46 (13.4248, 13.2702) -> (27.6248, 13.2702)
  line L47 (27.6248, 13.2702) -> (27.6248, -0.9298)
  line L48 (65.6248, 3.0702) -> (51.4248, 3.0702)
  line L49 (51.4248, 3.0702) -> (51.4248, 17.2702)
  line L50 (51.4248, 17.2702) -> (65.6248, 17.2702)
  line L51 (65.6248, 17.2702) -> (65.6248, 3.0702)
  line L52 (46.6248, 3.0702) -> (32.4248, 3.0702)
  line L53 (32.4248, 3.0702) -> (32.4248, 17.2702)
  line L54 (32.4248, 17.2702) -> (46.6248, 17.2702)
  line L55 (46.6248, 17.2702) -> (46.6248, 3.0702)
  line L56 (46.6248, -15.9298) -> (32.4248, -15.9298)
  line L57 (32.4248, -15.9298) -> (32.4248, -1.7298)
  line L58 (32.4248, -1.7298) -> (46.6248, -1.7298)
  line L59 (46.6248, -1.7298) -> (46.6248, -15.9298)
  line L60 (65.6248, -15.9298) -> (51.4248, -15.9298)
  line L61 (51.4248, -15.9298) -> (51.4248, -1.7298)
  line L62 (51.4248, -1.7298) -> (65.6248, -1.7298)
  line L63 (65.6248, -1.7298) -> (65.6248, -15.9298)
  line L64 (46.6248, -34.9298) -> (32.4248, -34.9298)
  line L65 (32.4248, -34.9298) -> (32.4248, -20.7298)
  line L66 (32.4248, -20.7298) -> (46.6248, -20.7298)
  line L67 (46.6248, -20.7298) -> (46.6248, -34.9298)
  line L68 (-29.3752, -51.9298) -> (-43.5752, -51.9298)
  line L69 (-43.5752, -51.9298) -> (-43.5752, -37.7298)
  line L70 (-43.5752, -37.7298) -> (-29.3752, -37.7298)
  line L71 (-29.3752, -37.7298) -> (-29.3752, -51.9298)
  line L72 (8.6248, -61.9298) -> (-5.5752, -61.9298)
  line L73 (-5.5752, -61.9298) -> (-5.5752, -47.7298)
  line L74 (-5.5752, -47.7298) -> (8.6248, -47.7298)
  line L75 (8.6248, -47.7298) -> (8.6248, -61.9298)
  line L76 (46.6248, -53.9298) -> (32.4248, -53.9298)
  line L77 (32.4248, -53.9298) -> (32.4248, -39.7298)
  line L78 (32.4248, -39.7298) -> (46.6248, -39.7298)
  line L79 (46.6248, -39.7298) -> (46.6248, -53.9298)
  line L80 (65.6248, -53.9298) -> (51.4248, -53.9298)
  line L81 (51.4248, -53.9298) -> (51.4248, -39.7298)
  line L82 (51.4248, -39.7298) -> (65.6248, -39.7298)
  line L83 (65.6248, -39.7298) -> (65.6248, -53.9298)
  line L84 (27.6248, -57.9298) -> (13.4248, -57.9298)
  line L85 (13.4248, -57.9298) -> (13.4248, -43.7298)
  line L86 (13.4248, -43.7298) -> (27.6248, -43.7298)
  line L87 (27.6248, -43.7298) -> (27.6248, -57.9298)
  line L88 (-10.3752, -54.9298) -> (-24.5752, -54.9298)
  line L89 (-24.5752, -54.9298) -> (-24.5752, -40.7298)
  line L90 (-24.5752, -40.7298) -> (-10.3752, -40.7298)
  line L91 (-10.3752, -40.7298) -> (-10.3752, -54.9298)
  line L92 (65.6248, -34.9298) -> (51.4248, -34.9298)
  line L93 (51.4248, -34.9298) -> (51.4248, -20.7298)
  line L94 (51.4248, -20.7298) -> (65.6248, -20.7298)
  line L95 (65.6248, -20.7298) -> (65.6248, -34.9298)
  line L96 (-53.9369, 44.8334) -> (-66.2388, 51.9258)
  line L97 (-66.2388, 51.9258) -> (-59.1465, 64.2278)
  line L98 (-59.1465, 64.2278) -> (-46.8445, 57.1354)
  line L99 (-46.8445, 57.1354) -> (-53.9369, 44.8334)
  line L100 (-38.6784, 33.259) -> (-50.9803, 40.3514)
  line L101 (-50.9803, 40.3514) -> (-43.8879, 52.6533)
  line L102 (-43.8879, 52.6533) -> (-31.586, 45.5609)
  line L103 (-31.586, 45.5609) -> (-38.6784, 33.259)
  line L104 (-22.218, 23.7692) -> (-34.52, 30.8616)
  line L105 (-34.52, 30.8616) -> (-27.4276, 43.1635)
  line L106 (-27.4276, 43.1635) -> (-15.1256, 36.0711)
  line L107 (-15.1256, 36.0711) -> (-22.218, 23.7692)
  line L108 (-44.7684, 55.9312) -> (-42.3648, 60.1005)
  line L109 (-42.3648, 60.1005) -> (-58.8251, 69.5903)
  line L110 (-58.8251, 69.5903) -> (-75.7872, 40.1691)
  line L111 (-75.7872, 40.1691) -> (-75.7872, 19.0772)
  line L112 (-75.7872, 19.0772) -> (-45.9752, 1.8653)
  line L113 (-45.9752, 1.8653) -> (-45.9752, -54.3298)
  line L114 (-45.9752, -54.3298) -> (-26.9752, -54.3298)
  line L115 (-26.9752, -54.3298) -> (-26.9752, -57.3298)
  line L116 (-26.9752, -57.3298) -> (-7.9752, -57.3298)
  line L117 (-7.9752, -57.3298) -> (-7.9752, -70.3298)
  line L118 (-7.9752, -70.3298) -> (68.0248, -70.3298)
  line L119 (68.0248, -70.3298) -> (68.0248, 19.6702)
  line L120 (68.0248, 19.6702) -> (30.0248, 19.6702)
  line L121 (30.0248, 19.6702) -> (30.0248, 15.6702)
  line L122 (30.0248, 15.6702) -> (-2.7791, 15.6702)
  line L123 (-2.7791, 15.6702) -> (-11.8477, 20.906)
  line L124 (-11.8477, 20.906) -> (-11.8477, 36.9516)
  line L125 (-11.8477, 36.9516) -> (-44.7684, 55.9312)
  line L126 (-66.9217, 51.7424) -> (-59.3299, 64.9107)
  line L127 (-59.3299, 64.9107) -> (-46.1616, 57.3188)
  line L128 (-46.1616, 57.3188) -> (-53.7535, 44.1505)
  line L129 (-53.7535, 44.1505) -> (-66.9217, 51.7424)
  line L130 (-30.9031, 45.7444) -> (-38.4949, 32.5761)
  line L131 (-38.4949, 32.5761) -> (-51.6632, 40.1679)
  line L132 (-51.6632, 40.1679) -> (-44.0714, 53.3362)
  line L133 (-44.0714, 53.3362) -> (-30.9031, 45.7444)
  line L134 (-35.2029, 30.6781) -> (-27.611, 43.8464)
  line L135 (-27.611, 43.8464) -> (-14.4427, 36.2546)
  line L136 (-14.4427, 36.2546) -> (-22.0346, 23.0863)
  line L137 (-22.0346, 23.0863) -> (-35.2029, 30.6781)
  line L138 (-44.0752, 4.5702) -> (-44.0752, 19.7702)
  line L139 (-44.0752, 19.7702) -> (-28.8752, 19.7702)
  line L140 (-28.8752, 19.7702) -> (-28.8752, 4.5702)
  line L141 (-28.8752, 4.5702) -> (-44.0752, 4.5702)
  line L142 (-25.0752, 1.5702) -> (-25.0752, 16.7702)
  line L143 (-25.0752, 16.7702) -> (-9.8752, 16.7702)
  line L144 (-9.8752, 16.7702) -> (-9.8752, 1.5702)
  line L145 (-9.8752, 1.5702) -> (-25.0752, 1.5702)
  line L146 (-6.0752, -5.4298) -> (-6.0752, 9.7702)
  line L147 (-6.0752, 9.7702) -> (9.1248, 9.7702)
  line L148 (9.1248, 9.7702) -> (9.1248, -5.4298)
  line L149 (9.1248, -5.4298) -> (-6.0752, -5.4298)
  line L150 (12.9248, -1.4298) -> (12.9248, 13.7702)
  line L151 (12.9248, 13.7702) -> (28.1248, 13.7702)
  line L152 (28.1248, 13.7702) -> (28.1248, -1.4298)
  line L153 (28.1248, -1.4298) -> (12.9248, -1.4298)
  line L154 (47.1248, 2.5702) -> (31.9248, 2.5702)
  line L155 (31.9248, 2.5702) -> (31.9248, 17.7702)
  line L156 (31.9248, 17.7702) -> (47.1248, 17.7702)
  line L157 (47.1248, 17.7702) -> (47.1248, 2.5702)
  line L158 (-28.8752, -14.4298) -> (-44.0752, -14.4298)
  line L159 (-44.0752, -14.4298) -> (-44.0752, 0.7702)
  line L160 (-44.0752, 0.7702) -> (-28.8752, 0.7702)
  line L161 (-28.8752, 0.7702) -> (-28.8752, -14.4298)
  line L162 (66.1248, 2.5702) -> (50.9248, 2.5702)
  line L163 (50.9248, 2.5702) -> (50.9248, 17.7702)
  line L164 (50.9248, 17.7702) -> (66.1248, 17.7702)
  line L165 (66.1248, 17.7702) -> (66.1248, 2.5702)
  line L166 (-25.0752, -17.4298) -> (-25.0752, -2.2298)
  line L167 (-25.0752, -2.2298) -> (-9.8752, -2.2298)
  line L168 (-9.8752, -2.2298) -> (-9.8752, -17.4298)
  line L169 (-9.8752, -17.4298) -> (-25.0752, -17.4298)
  line L170 (-6.0752, -24.4298) -> (-6.0752, -9.2298)
  line L171 (-6.0752, -9.2298) -> (9.1248, -9.2298)
  line L172 (9.1248, -9.2298) -> (9.1248, -24.4298)
  line L173 (9.1248, -24.4298) -> (-6.0752, -24.4298)
  line L174 (12.9248, -20.4298) -> (12.9248, -5.2298)
  line L175 (12.9248, -5.2298) -> (28.1248, -5.2298)
  line L176 (28.1248, -5.2298) -> (28.1248, -20.4298)
  line L177 (28.1248, -20.4298) -> (12.9248, -20.4298)
  line L178 (31.9248, -16.4298) -> (31.9248, -1.2298)
  line L179 (31.9248, -1.2298) -> (47.1248, -1.2298)
  line L180 (47.1248, -1.2298) -> (47.1248, -16.4298)
  line L181 (47.1248, -16.4298) -> (31.9248, -16.4298)
  line L182 (50.9248, -16.4298) -> (50.9248, -1.2298)
  line L183 (50.9248, -1.2298) -> (66.1248, -1.2298)
  line L184 (66.1248, -1.2298) -> (66.1248, -16.4298)
  line L185 (66.1248, -16.4298) -> (50.9248, -16.4298)
  line L186 (50.9248, -35.4298) -> (50.9248, -20.2298)
  line L187 (50.9248, -20.2298) -> (66.1248, -20.2298)
  line L188 (66.1248, -20.2298) -> (66.1248, -35.4298)
  line L189 (66.1248, -35.4298) -> (50.9248, -35.4298)
  line L190 (31.9248, -35.4298) -> (31.9248, -20.2298)
  line L191 (31.9248, -20.2298) -> (47.1248, -20.2298)
  line L192 (47.1248, -20.2298) -> (47.1248, -35.4298)
  line L193 (47.1248, -35.4298) -> (31.9248, -35.4298)
  line L194 (12.9248, -39.4298) -> (12.9248, -24.2298)
  line L195 (12.9248, -24.2298) -> (28.1248, -24.2298)
  line L196 (28.1248, -24.2298) -> (28.1248, -39.4298)
  line L197 (28.1248, -39.4298) -> (12.9248, -39.4298)
  line L198 (-6.0752, -43.4298) -> (-6.0752, -28.2298)
  line L199 (-6.0752, -28.2298) -> (9.1248, -28.2298)
  line L200 (9.1248, -28.2298) -> (9.1248, -43.4298)
  line L201 (9.1248, -43.4298) -> (-6.0752, -43.4298)
  line L202 (-25.0752, -36.4298) -> (-25.0752, -21.2298)
  line L203 (-25.0752, -21.2298) -> (-9.8752, -21.2298)
  line L204 (-9.8752, -21.2298) -> (-9.8752, -36.4298)
  line L205 (-9.8752, -36.4298) -> (-25.0752, -36.4298)
  line L206 (-44.0752, -33.4298) -> (-44.0752, -18.2298)
  line L207 (-44.0752, -18.2298) -> (-28.8752, -18.2298)
  line L208 (-28.8752, -18.2298) -> (-28.8752, -33.4298)
  line L209 (-28.8752, -33.4298) -> (-44.0752, -33.4298)
  line L210 (-44.0752, -52.4298) -> (-44.0752, -37.2298)
  line L211 (-44.0752, -37.2298) -> (-28.8752, -37.2298)
  line L212 (-28.8752, -37.2298) -> (-28.8752, -52.4298)
  line L213 (-28.8752, -52.4298) -> (-44.0752, -52.4298)
  line L214 (-25.0752, -55.4298) -> (-25.0752, -40.2298)
  line L215 (-25.0752, -40.2298) -> (-9.8752, -40.2298)
  line L216 (-9.8752, -40.2298) -> (-9.8752, -55.4298)
  line L217 (-9.8752, -55.4298) -> (-25.0752, -55.4298)
  line L218 (-6.0752, -62.4298) -> (-6.0752, -47.2298)
  line L219 (-6.0752, -47.2298) -> (9.1248, -47.2298)
  line L220 (9.1248, -47.2298) -> (9.1248, -62.4298)
  line L221 (9.1248, -62.4298) -> (-6.0752, -62.4298)
  line L222 (12.9248, -58.4298) -> (12.9248, -43.2298)
  line L223 (12.9248, -43.2298) -> (28.1248, -43.2298)
  line L224 (28.1248, -43.2298) -> (28.1248, -58.4298)
  line L225 (28.1248, -58.4298) -> (12.9248, -58.4298)
  line L226 (31.9248, -54.4298) -> (31.9248, -39.2298)
  line L227 (31.9248, -39.2298) -> (47.1248, -39.2298)
  line L228 (47.1248, -39.2298) -> (47.1248, -54.4298)
  line L229 (47.1248, -54.4298) -> (31.9248, -54.4298)
  line L230 (50.9248, -54.4298) -> (50.9248, -39.2298)
  line L231 (50.9248, -39.2298) -> (66.1248, -39.2298)
  line L232 (66.1248, -39.2298) -> (66.1248, -54.4298)
  line L233 (66.1248, -54.4298) -> (50.9248, -54.4298)
  line L234 (-57.0872, 20.2441) -> (-69.4872, 20.2441)
  line L235 (-69.4872, 20.2441) -> (-69.4872, 32.3441)
  line L236 (-69.4872, 32.3441) -> (-57.0872, 32.3441)
  line L237 (-57.0872, 32.3441) -> (-57.0872, 20.2441)
  line L238 (-71.0372, 33.2941) -> (-55.0372, 33.2941)
  line L239 (-55.0372, 33.2941) -> (-55.0372, 19.2941)
  line L240 (-55.0372, 19.2941) -> (-71.0372, 19.2941)
  line L241 (-71.0372, 19.2941) -> (-71.0372, 33.2941)
  dimension "d82" = -0.5
  dimension "d83" = -0.5
  dimension "d84" = -0.5
  dimension "d85" = -0.5
  dimension "d86" = -0.5
  dimension "d87" = -0.5
  dimension "d88" = -0.5
  dimension "d89" = -0.5
  dimension "d90" = -0.5
  dimension "d91" = -0.5
  dimension "d92" = -0.5
  dimension "d93" = -0.5
  dimension "d94" = -0.5
  dimension "d95" = -0.5
  dimension "d96" = -0.5
  dimension "d97" = -0.5
  dimension "d98" = -0.5
  dimension "d99" = -0.5
  dimension "d100" = -0.5
  dimension "d101" = -0.5
  dimension "d102" = -0.5
  dimension "d103" = -0.5
  dimension "d104" = -0.5
  dimension "d105" = -0.5
  dimension "d106" = -0.5
  dimension "d107" = -0.5
  dimension "d108" = -0.5
  dimension "d113" = 16
  dimension "d114" = 14
  dimension "d116" = 12.4
  dimension "d117" = 12.1
  dimension "d118" = 0.95
  dimension "d119" = 2.05
  constraint horizontal L238
  constraint vertical L239
  constraint horizontal L240
  constraint vertical L241
  measures "d113" distance of L238.start L238.end
  measures "d114" distance of L238.start L240.end
  measures "d116" distance of L235 L237
  measures "d117" distance of L234 L236
  measures "d118" distance of L236 L238
  measures "d119" distance of L237 L239
extrude "Extrude4" cut sketch "Sketch6" against normal blind 1.3 contours L126 L127 L128 L129 | L130 L131 L132 L133 | L134 L135 L136 L137 | L138 L139 L140 L141 | L142 L143 L144 L145 | L146 L147 L148 L149 | L150 L151 L152 L153 | L154 L155 L156 L157 | L158 L159 L160 L161 | L162 L163 L164 L165 | L166 L167 L168 L169 | L170 L171 L172 L173 | L174 L175 L176 L177 | L178 L179 L180 L181 | L182 L183 L184 L185 | L186 L187 L188 L189 | L190 L191 L192 L193 | L194 L195 L196 L197 | L198 L199 L200 L201 | L202 L203 L204 L205 | L206 L207 L208 L209 | L210 L211 L212 L213 | L214 L215 L216 L217 | L218 L219 L220 L221 | L222 L223 L224 L225 | L226 L227 L228 L229 | L230 L231 L232 L233 bodies 1
extrude "Extrude5" cut sketch "Sketch6" against normal blind 1.5 contours L238 L239 L240 L241 bodies 1